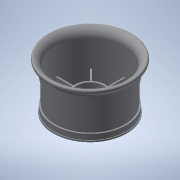
# Autodesk Inventor part: 風鼓本體
Saved by Autodesk Inventor 2020 (Build 240168000, 168)
## iProperties
Created: 2017-11-27
Part Number: 風鼓本體
Material: 一般
Document SubType Name: Modeling
Designer: USER
Density: 1 g/cm^3
Appearance: Default
Author: USER
Autodesk Inventor part; units mm, degrees
ref_plane "YZ Plane" through (0, 0, 0) normal (1, 0, 0) x (0, 1, 0)
ref_plane "XZ Plane" through (0, 0, 0) normal (0, 1, 0) x (-1, 0, 0)
ref_plane "XY Plane" through (0, 0, 0) normal (0, 0, 1) x (1, 0, 0)
sketch "草圖1" plane through (0, 0, 0) normal (0, 0, 1) x (1, 0, 0)
  circle A0 centre (0, 0) radius 26.5
  dimension "d0" = 53
  constraints: 1 centre point, 1 coincident
  measures "d0" diameter of A0
extrude "擠出1" add sketch "草圖1" along normal blind 35.5
sketch "草圖2" plane through (0, 0, 35.5) normal (0, 0, 1) x (1, 0, 0)
  circle A0 centre (0, 0) radius 30.65
  dimension "d3" = 61.3
  constraints: 1 centre point, 1 coincident
  measures "d3" diameter of A0
extrude "擠出2" add sketch "草圖2" against normal blind 7
sketch "草圖3" plane through (0, 0, 0) normal (0, 1, 0) x (-1, 0, 0)
  line L0 (-30.65, 35.5) -> (-30.65, 28.5) projected
  line L1 (-30.65, 28.5) -> (30.65, 28.5) projected
  circle A0 centre (-30.65, 28.5) radius 4.15
  line L2 (-26.5, 0) -> (-26.5, 28.5) projected
  line L3 (0, -7.1) -> (0, 42.6) projected
  point P0 (0, 0)
  constraints: 1 centre point, 1 coincident, 1 tangent
revolve "迴轉1" cut sketch "草圖3" angle 360 about axis through (0, 0, -10) along (0, 0, 1)
sketch "草圖4" plane through (0, 0, 0) normal (0, 0, -1) x (-1, 0, 0)
  circle A0 centre (0, 0) radius 27
  dimension "d8" = 54
  constraints: 1 centre point, 1 coincident
  measures "d8" diameter of A0
extrude "擠出3" add sketch "草圖4" against normal blind 1
sketch "草圖5" plane through (0, 0, 0) normal (0, 1, 0) x (-1, 0, 0)
  line L0 (27, 1) -> (-27, 1) projected
  line L1 (-26.5, 1) -> (-26.5, 28.5) projected
  line L2 (-26.5, 8) -> (-25.5, 8)
  line L3 (-25.5, 8) -> (-25.5, 5)
  line L4 (-25.5, 5) -> (-26.5, 5)
  line L5 (-26.5, 5) -> (-26.5, 8)
  line L6 (0, -5.7) -> (0, 34.2) projected
  line L7 (-26.5, 8) -> (-25.85, 8)
  line L8 (-25.85, 8) -> (-25.85, 22.7)
  line L9 (-25.85, 22.7) -> (-26.5, 22.7)
  line L10 (-26.5, 22.7) -> (-26.5, 8)
  line L11 (26.5, 1) -> (26.5, 28.5) projected
  point P0 (0, 0)
  dimension "d11" = 4
  dimension "d12" = 3
  dimension "d13" = 1
  dimension "d15" = 14.7
  dimension "d16" = 0.65
  dimension "d44" = 52.35
  dimension "d45" = 53
  constraints: 16 end point, 3 perpendicular, 2 horizontal, 2 parallel, 2 point on line, 1 collinear
  measures "d11" distance between parallel lines of L0 L4
  measures "d12" distance of L2.end L3.end
  measures "d13" distance of L3.end L4.end
  measures "d15" distance of L7.end L8.end
  measures "d16" distance of L8.end L9.end
  measures "d44" distance between parallel lines of L11 L8
  measures "d45" distance between parallel lines of L11 L1
revolve "迴轉2" cut sketch "草圖5" angle 360 about axis through (0, 0, -10) along (0, 0, 1)
sketch "草圖6" plane through (0, 0, 0) normal (0, 0, -1) x (-1, 0, 0)
  circle A0 centre (0, 0) radius 25
  dimension "d17" = 50
  constraints: 1 centre point, 1 coincident
  measures "d17" diameter of A0
extrude "擠出4" cut sketch "草圖6" against normal through all
fillet "圓角1" radius 6 1 edges at (25, 0, 35.5)
fillet "圓角2" radius 1 3 edges at (0, 30.65, 35.5) (0, -30.65, 35.5) (-30.65, 0, 32.65)
sketch "草圖7" plane through (0, 0, 0) normal (0, 0, -1) x (-1, 0, 0)
  circle A0 centre (0, 0) radius 25 projected
extrude "擠出5" add sketch "草圖7" along normal blind 7
sketch "草圖8" plane through (0, 0, 0) normal (0, 1, 0) x (-1, 0, 0)
  line L0 (-11.25, -3.7274) -> (-11.25, -14.6883) construction
  line L1 (25, 0) -> (-25, 0) projected
  line L2 (-25, 0) -> (-25, -7) projected
  line L3 (-25, 0) -> (-11.25, -7)
  line L4 (-25, -7) -> (25, -7) projected
  line L5 (-25, 0) -> (-25, -7)
  line L6 (27, 0) -> (-27, 0) projected
  line L7 (-25, -7) -> (-11.25, -7)
  line L8 (0, -17.626) -> (0, 2.9377) projected
  point P0 (0, 0)
  dimension "d24" = 11.25
  constraints: 8 end point, 2 perpendicular, 2 point on line, 1 vertical
  measures "d24" distance from line of L0 point (0, 0)
revolve "迴轉3" cut sketch "草圖8" angle 360 about axis through (0, 0, -10) along (0, 0, 1) contours L3 L4 L2
sketch "草圖9" plane through (0, 0, -7) normal (0, 0, -1) x (-1, 0, 0)
  circle A0 centre (0, 0) radius 10
  dimension "d26" = 20
  constraints: 1 centre point, 1 coincident
  measures "d26" diameter of A0
extrude "擠出6" cut sketch "草圖9" against normal through all
sketch "草圖10" plane through (0, 0, 0) normal (0, 0, -1) x (-1, 0, 0)
  circle A0 centre (0, 0) radius 25 projected
  line L0 (0, 0) -> (-42.0173, 0)
  line L1 (-17.6777, 17.6777) -> (0, 0) construction
  circle A1 centre (0, 0) radius 11.25 projected
  line L2 (-11.25, 0) -> (-25, 0)
  arc A2 (-8.6306, 7.2164) -> (-11.25, 0) centre (0, 0) ccw
  arc A3 (-17.6777, 17.6777) -> (-25, 0) centre (0, 0) ccw
  line L3 (-8.6306, 7.2164) -> (-18.3706, 16.9564)
  point P0 (-17.6777, -17.6777)
  point P1 (0, -25)
  point P2 (17.6777, -17.6777)
  point P3 (25, 0)
  point P4 (17.6777, 17.6777)
  point P5 (0, 25)
  point P6 (-7.955, 7.955)
  dimension "d31" = 360
  dimension "d36" = 1
  constraints: 8 end point, 5 point on circle, 3 point on line, 2 centre point, 2 coincident, 2 horizontal, 2 horizontal alignment, 1 parallel, 13 other
  measures "d36" distance between parallel lines of L3 L1
extrude "擠出7" cut sketch "草圖10" along normal through all contours A0 L3 A1 L0 picked at (-20.0602, 2.912)
pattern_circular "環形陣列1" count 8 over 360 about axis through (0, 0, -10) along (0, 0, 1) of "擠出7"
sketch "草圖11" plane through (0, 0, 0) normal (0, 0, 1) x (1, 0, 0)
  line L0 (11.2055, -1) -> (24.98, -1) projected
  arc A0 (24.98, -1) -> (25, 0) centre (0, 0) ccw projected
  line L1 (25, 0) -> (11.25, 0) projected
  arc A1 (11.25, 0) -> (8.6306, 7.2164) centre (0, 0) ccw projected
  line L2 (8.6306, 7.2164) -> (18.3706, 16.9564) projected
  arc A2 (18.3706, 16.9564) -> (17.6777, 17.6777) centre (0, 0) ccw projected
  line L3 (17.6777, 17.6777) -> (7.955, 7.955) projected
  arc A3 (7.955, 7.955) -> (1, 11.2055) centre (0, 0) ccw projected
  line L4 (1, 11.2055) -> (1, 24.98) projected
  arc A4 (1, 24.98) -> (0, 25) centre (0, 0) ccw projected
  line L5 (0, 25) -> (0, 11.25) projected
  arc A5 (0, 11.25) -> (-7.2164, 8.6306) centre (0, 0) ccw projected
  line L6 (-7.2164, 8.6306) -> (-16.9564, 18.3706) projected
  arc A6 (-16.9564, 18.3706) -> (-17.6777, 17.6777) centre (0, 0) ccw projected
  line L7 (-17.6777, 17.6777) -> (-7.955, 7.955) projected
  arc A7 (-7.955, 7.955) -> (-11.2055, 1) centre (0, 0) ccw projected
  line L8 (-11.2055, 1) -> (-24.98, 1) projected
  arc A8 (-24.98, 1) -> (-25, 0) centre (0, 0) ccw projected
  line L9 (-25, 0) -> (-11.25, 0) projected
  arc A9 (-11.25, 0) -> (-8.6306, -7.2164) centre (0, 0) ccw projected
  line L10 (-8.6306, -7.2164) -> (-18.3706, -16.9564) projected
  arc A10 (-18.3706, -16.9564) -> (-17.6777, -17.6777) centre (0, 0) ccw projected
  line L11 (-17.6777, -17.6777) -> (-7.955, -7.955) projected
  arc A11 (-7.955, -7.955) -> (-1, -11.2055) centre (0, 0) ccw projected
  line L12 (-1, -11.2055) -> (-1, -24.98) projected
  arc A12 (-1, -24.98) -> (0, -25) centre (0, 0) ccw projected
  line L13 (0, -25) -> (0, -11.25) projected
  arc A13 (0, -11.25) -> (7.2164, -8.6306) centre (0, 0) ccw projected
  line L14 (7.2164, -8.6306) -> (16.9564, -18.3706) projected
  arc A14 (16.9564, -18.3706) -> (17.6777, -17.6777) centre (0, 0) ccw projected
  line L15 (17.6777, -17.6777) -> (7.955, -7.955) projected
  arc A15 (7.955, -7.955) -> (11.2055, -1) centre (0, 0) ccw projected
  circle A16 centre (0, 0) radius 10 projected
extrude "擠出8" add sketch "草圖11" along normal blind 10
sketch "草圖12" plane through (0, 0, 10) normal (0, 0, 1) x (1, 0, 0)
  circle A0 centre (0, 0) radius 11.25
  circle A1 centre (0, 0) radius 10
  arc A2 (0, 11.25) -> (-7.2164, 8.6306) centre (0, 0) ccw projected
  circle A3 centre (0, 0) radius 10 projected
  constraints: 2 centre point, 2 coincident, 2 concentric
extrude "擠出9" add sketch "草圖12" along normal blind 2
